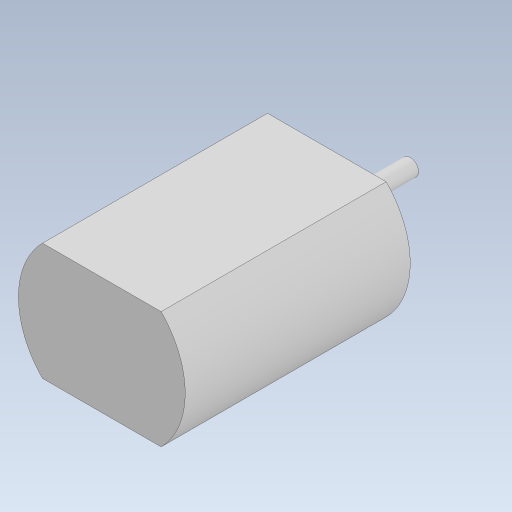
# Autodesk Inventor part: motor 12v
Saved by Autodesk Inventor 2023 (Build 270158000, 158)
## iProperties
Created: 2023-03-23
Part Number: motor 12v
Material: Generic
Document SubType Name: Modeling
Designer: dverd
Density: 1 g/cm^3
Appearance: Default
Author: dverd
Autodesk Inventor part; units mm, degrees
ref_plane "YZ Plane" through (0, 0, 0) normal (1, 0, 0) x (0, 1, 0)
ref_plane "XZ Plane" through (0, 0, 0) normal (0, 1, 0) x (-1, 0, 0)
ref_plane "XY Plane" through (0, 0, 0) normal (0, 0, 1) x (1, 0, 0)
sketch "Sketch1" plane through (0, 0, 0) normal (0, 0, 1) x (1, 0, 0)
  circle A0 centre (0, 0) radius 10
  line L0 (0, 10) -> (0, 9)
  line L1 (-7.116, 7.0259) -> (7.116, 7.0259)
  line L2 (7.116, -7.0259) -> (-7.116, -7.0259)
  dimension "d0" = 20
  dimension "d7" = 14.0518
  constraints: 6 end point, 5 point on circle, 2 parallel, 1 centre point, 1 coincident, 1 horizontal, 1 vertical
  measures "d0" diameter of A0
  measures "d7" distance between parallel lines of L2 L1
extrude "Extrusion1" add sketch "Sketch1" against normal blind 27 contours A0 L2 L1
sketch "Sketch2" plane through (0, 0, -27) normal (0, 0, -1) x (0, -1, 0)
  circle A0 centre (0, 0) radius 1
  dimension "d4" = 2
  constraints: 1 centre point, 1 coincident
  measures "d4" diameter of A0
extrude "Extrusion2" add sketch "Sketch2" along normal blind 10
body "Solid1"
